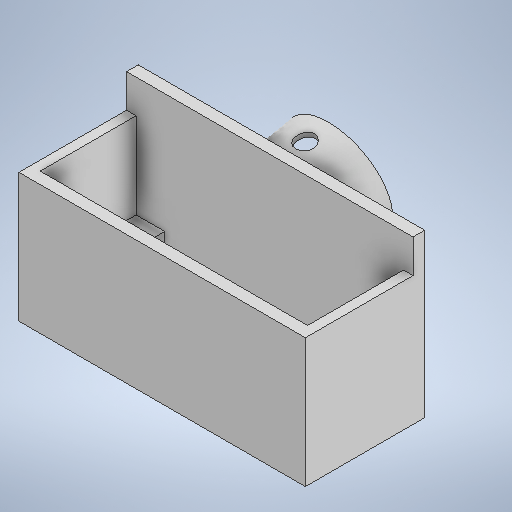
# Autodesk Inventor part: Attache servomoteur
Saved by Autodesk Inventor 2026.2 (Build 302298010, 298A)
## iProperties
Created: 2026-03-22
Part Number: Attache servomoteur
Material: Générique
Document SubType Name: Modeling
Designer: Genon
Density: 1 g/cm^3
Appearance: Par défaut
Author: Genon
Autodesk Inventor part; units mm, degrees
ref_plane "YZ Plane" through (0, 0, 0) normal (1, 0, 0) x (0, 1, 0)
sketch "Esquisse1" plane through (0, 0, 0) normal (0, 1, 0) x (-1, 0, 0)
  line L0 (0, 0) -> (30, 0)
  line L1 (30, 0) -> (30, 25)
  line L2 (30, 25) -> (-30, 25)
  line L3 (-30, 25) -> (-30, 0)
  line L4 (-30, 0) -> (0, 0)
  line L5 (0, 0) -> (0, 2.45)
  line L6 (0, 2.45) -> (28, 2.45)
  line L7 (28, 2.45) -> (28, 22.55)
  line L8 (28, 22.55) -> (-28, 22.55)
  line L9 (-28, 22.55) -> (-28, 2.45)
  line L10 (-28, 2.45) -> (0, 2.45)
  dimension "d0" = 30
  dimension "d1" = 25
  dimension "d2" = 60
  dimension "d3" = 30
  dimension "d4" = 2.45
  dimension "d5" = 28
  dimension "d7" = 20.1
  dimension "d8" = 56
  constraints: 22 end point, 7 perpendicular, 2 vertical, 1 horizontal, 1 parallel, 1 point on line
  measures "d0" distance of L0.start L0.end
  measures "d1" distance of L0.end L1.end
  measures "d2" distance of L1.end L2.end
  measures "d3" distance of L3.end L0.start
  measures "d4" distance of L0.start L5.end
  measures "d5" distance of L5.end L6.end
  measures "d7" distance of L6.end L7.end
  measures "d8" distance of L7.end L8.end
extrude "Extrusion1" add sketch "Esquisse1" along normal blind 27
ref_plane "Plan de construction1" through (0, 0, 0) normal (0, 0.2046669, -0.9788317) x (1, 0, 0)
sketch "Esquisse10" plane through (0, 27, 0) normal (0, 1, 0) x (1, 0, 0)
  line L0 (-30, 0) -> (-30, -25) projected
  line L1 (30, -25) -> (30, 0) projected
  line L2 (-30, 0) -> (30, 0)
  line L3 (30, 0) -> (30, -2.45)
  line L4 (30, -2.45) -> (-30, -2.45)
  line L5 (-30, -2.45) -> (-30, 0)
  point P0 (0, 0)
  point P1 (30, 0)
  dimension "d67" = 2.45
  constraints: 8 end point, 2 parallel, 1 horizontal, 1 perpendicular, 1 point on line
  measures "d67" distance of L2.end L3.end
extrude "Extrusion8" add sketch "Esquisse10" along normal blind 7
sketch "Esquisse2" plane through (0, 0, 0) normal (0, 0.2046669, -0.9788317) x (1, 0, 0)
  line L0 (0, 0) -> (0, -20)
  circle A0 centre (0, -20) radius 10
  circle A1 centre (0, -20) radius 11
  dimension "d12" = 20
  dimension "d13" = 20
  dimension "d14" = 22
  constraints: 2 centre point, 2 coincident, 2 end point, 1 vertical
  measures "d12" distance of L0.start L0.end
  measures "d13" diameter of A0
  measures "d14" diameter of A1
extrude "Extrusion2" add sketch "Esquisse2" along normal blind 16.5
sketch "Esquisse3" plane through (0, 27, 0) normal (0, 1, 0) x (1, 0, 0)
  line L0 (-28, -22.55) -> (-28, -2.45) projected
  line L1 (28, -22.55) -> (-28, -22.55) projected
  line L2 (-28, -2.45) -> (28, -2.45) projected
  line L3 (28, -2.45) -> (28, -22.55) projected
  point P0 (0, 0)
extrude "Extrusion3" cut sketch "Esquisse3" against normal through all
ref_plane "Plan de construction2" through (0, 1.3303, -6.3624) normal (0, 0.2046669, -0.9788317) x (1, 0, 0)
sketch "Esquisse4" plane through (0, 1.3303, -6.3624) normal (0, 0.2046669, -0.9788317) x (1, 0, 0)
  circle A0 centre (0, -20) radius 10 projected
  point P0 (0, 0)
extrude "Extrusion4" add sketch "Esquisse4" against normal blind 2
ref_plane "Plan de construction3" through (30, 0, 0) normal (0, -0.9788317, -0.2046669) x (-1, 0, 0)
sketch "Esquisse5" plane through (30, 0, 0) normal (0, -0.9788317, -0.2046669) x (-1, 0, 0)
  line L0 (41, 16.5) -> (19, 16.5) projected
  line L1 (30, 16.5) -> (30, 11.5)
  point P0 (30, 0)
  dimension "d23" = 5
  constraints: 2 end point, 1 coincident, 1 midpoint, 1 vertical
  measures "d23" distance of L1.start L1.end
hole "Perçage1" at (0, 2.3537, -11.2566) direction (0, 0.9788317, 0.2046669) diameter 4 end through all
sketch "Esquisse6" plane through (0, 0, 0) normal (0, -1, 0) x (1, 0, 0)
  line L0 (28, 2.45) -> (28, 22.55) projected
  line L1 (-28, 22.55) -> (-28, 2.45) projected
  line L2 (28, 22.55) -> (22, 22.55)
  line L3 (28, 22.55) -> (-28, 22.55) projected
  line L4 (22, 22.55) -> (22, 2.45)
  line L5 (22, 2.45) -> (28, 2.45)
  line L6 (-28, 22.55) -> (-22, 22.55)
  line L7 (-22, 22.55) -> (-22, 2.45)
  line L8 (-22, 2.45) -> (-28, 2.45)
  point P0 (0, 0)
  dimension "d31" = 6
  dimension "d32" = 6
  constraints: 12 end point, 4 perpendicular, 3 point on line
  measures "d31" distance of L0.end L2.end
  measures "d32" distance of L1.start L6.end
extrude "Extrusion5" add sketch "Esquisse6" against normal blind 9
sketch "Esquisse7" plane through (0, 9, 0) normal (0, 1, 0) x (1, 0, 0)
  line L0 (-28, -22.55) -> (-28, -2.45) projected
  line L1 (-28, -12.5) -> (-25, -12.5)
  line L2 (-25, -12.5) -> (-25, -17.5)
  line L3 (-25, -12.5) -> (-25, -7.5)
  line L4 (28, -2.45) -> (28, -22.55) projected
  line L5 (28, -22.55) -> (28, -12.5)
  line L6 (28, -12.5) -> (25, -12.5)
  line L7 (25, -12.5) -> (25, -7.5)
  line L8 (22, -22.55) -> (22, -2.45) projected
  line L9 (25, -12.5) -> (25, -17.5)
  point P0 (0, 0)
  dimension "d35" = 3
  dimension "d36" = 5
  dimension "d37" = 5
  dimension "d38" = 3
  dimension "d39" = 5
  dimension "d41" = 5
  constraints: 14 end point, 4 coincident, 3 perpendicular, 2 midpoint, 2 vertical, 1 horizontal
  measures "d35" distance of L1.start L1.end
  measures "d36" distance of L1.end L2.end
  measures "d37" distance of L1.end L3.end
  measures "d38" distance of L5.end L6.end
  measures "d39" distance of L6.end L7.end
  measures "d41" distance of L6.end L9.end
hole "Perçage2" at (-25, 9, 17.5) at (-25, 9, 7.5) at (25, 9, 17.5) at (25, 9, 7.5) direction (0, -1, 0) diameter 3.242 depth 11.8 tip angle 118 thread size "M4x0.7" class "6H" standard "ISO Metric profile"
sketch "Esquisse8" plane through (0, 9, 0) normal (0, 1, 0) x (1, 0, 0)
  line L0 (-22, -22.55) -> (-22, -2.45) projected
  line L1 (-28, -22.55) -> (-28, -2.45) projected
  line L2 (-28, -12.5) -> (-28, -11.5)
  line L3 (-28, -11.5) -> (-22, -11.5)
  line L4 (-28, -12.5) -> (-28, -13.5)
  line L5 (-28, -13.5) -> (-22, -13.5)
  line L6 (-22, -11.5) -> (-22, -13.5)
  line L7 (22, -2.45) -> (22, -22.55) projected
  line L8 (28, -2.45) -> (28, -22.55) projected
  line L9 (28, -22.55) -> (28, -12.5)
  line L10 (28, -12.5) -> (28, -11.5)
  line L11 (22, -11.5) -> (28, -11.5)
  line L12 (22, -11.5) -> (22, -13.5)
  line L13 (22, -13.5) -> (28, -13.5)
  point P0 (0, 0)
  point P1 (28, -12.5)
  point P2 (28, -13.5)
  dimension "d49" = 1
  dimension "d50" = 1
  dimension "d54" = 10.05
  dimension "d55" = 6
  dimension "d56" = 2
  dimension "d57" = 1
  constraints: 20 end point, 8 point on line, 5 perpendicular, 3 midpoint
  measures "d49" distance of L2.start L2.end
  measures "d50" distance of L2.start L4.end
  measures "d54" distance of L8.end L9.end
  measures "d55" distance of L11.start L10.end
  measures "d56" distance of L11.start L12.end
  measures "d57" distance of L13.end point (28, -12.5)
extrude "Extrusion6" cut sketch "Esquisse8" against normal blind 2
sketch "Esquisse11" plane through (0, 34, 0) normal (0, 1, 0) x (1, 0, 0)
  ellipse E0 centre (0, 31.4094) end of major axis (0, 85.1552) minor radius 11 (-8.5426, -2.45) -> (-7.9677, -5.6455) ccw projected
  ellipse E1 centre (0, -4.0933) end of major axis (11, -4.0933) minor radius 2.2513 (-7.9677, -5.6455) -> (7.9677, -5.6455) ccw projected
  ellipse E2 centre (0, 31.4094) end of major axis (0, 85.1552) minor radius 11 (7.9677, -5.6455) -> (8.5426, -2.45) ccw projected
  line L0 (-8.5426, -2.45) -> (8.5426, -2.45) projected
  point P0 (0, 0)
  constraints: 3 other
extrude "Extrusion9" cut sketch "Esquisse11" against normal blind 10
